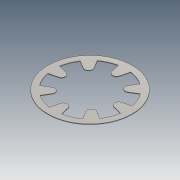
# Autodesk Inventor part: Arruela do parafuso da tampa
Saved by Autodesk Inventor 2016 (Build 200138000, 138)
## iProperties
Created: 2018-12-06
Part Number: Arruela do parafuso da tampa
Material: Generic
Document SubType Name: Modeling
Designer: Aluno
Density: 1 g/cm^3
Appearance: Galvanized
Author: Aluno
Autodesk Inventor part; units mm, degrees
ref_plane "YZ Plane" through (0, 0, 0) normal (1, 0, 0) x (0, 1, 0)
ref_plane "XZ Plane" through (0, 0, 0) normal (0, 1, 0) x (-1, 0, 0)
ref_plane "XY Plane" through (0, 0, 0) normal (0, 0, 1) x (1, 0, 0)
sketch "Sketch1" plane through (0, 0, 0) normal (0, 0, 1) x (1, 0, 0)
  circle A0 centre (0, 0) radius 7
  line L0 (0.1571, -3.914) -> (0.6571, -3.914)
  line L1 (0.6571, -3.914) -> (-0.3428, -3.914)
  line L2 (-0.3428, -3.914) -> (-0.8427, -5.9405)
  line L3 (0.6571, -3.914) -> (1.157, -5.8874)
  line L4 (2.5252, -3.01) -> (3.6047, -4.7964)
  line L5 (3.2322, -2.303) -> (4.9811, -3.3449)
  line L6 (2.8787, -2.6565) -> (3.2322, -2.303)
  line L7 (3.2322, -2.303) -> (2.5252, -3.01)
  line L8 (3.914, -0.3428) -> (5.9405, -0.8427)
  line L9 (3.914, 0.6571) -> (5.8874, 1.157)
  line L10 (3.914, 0.1571) -> (3.914, 0.6571)
  line L11 (3.914, 0.6571) -> (3.914, -0.3428)
  line L12 (3.01, 2.5252) -> (4.7964, 3.6047)
  line L13 (2.303, 3.2322) -> (3.3449, 4.9811)
  line L14 (2.6565, 2.8787) -> (2.303, 3.2322)
  line L15 (2.303, 3.2322) -> (3.01, 2.5252)
  line L16 (0.3428, 3.914) -> (0.8427, 5.9405)
  line L17 (-0.6571, 3.914) -> (-1.157, 5.8874)
  line L18 (-0.1571, 3.914) -> (-0.6571, 3.914)
  line L19 (-0.6571, 3.914) -> (0.3428, 3.914)
  line L20 (-2.5252, 3.01) -> (-3.6047, 4.7964)
  line L21 (-3.2322, 2.303) -> (-4.9811, 3.3449)
  line L22 (-2.8787, 2.6565) -> (-3.2322, 2.303)
  line L23 (-3.2322, 2.303) -> (-2.5252, 3.01)
  line L24 (-3.914, 0.3428) -> (-5.9405, 0.8427)
  line L25 (-3.914, -0.6571) -> (-5.8874, -1.157)
  line L26 (-3.914, -0.1571) -> (-3.914, -0.6571)
  line L27 (-3.914, -0.6571) -> (-3.914, 0.3428)
  line L28 (-3.01, -2.5252) -> (-4.7964, -3.6047)
  line L29 (-2.303, -3.2322) -> (-3.3449, -4.9811)
  line L30 (-2.6565, -2.8787) -> (-2.303, -3.2322)
  line L31 (-2.303, -3.2322) -> (-3.01, -2.5252)
  arc A1 (-4.9811, 3.3449) -> (-5.9405, 0.8427) centre (0, 0) ccw
  arc A2 (-1.157, 5.8874) -> (-3.6047, 4.7964) centre (0, 0) ccw
  arc A3 (3.3449, 4.9811) -> (0.8427, 5.9405) centre (0, 0) ccw
  arc A4 (5.8874, 1.157) -> (4.7964, 3.6047) centre (0, 0) ccw
  arc A5 (4.9811, -3.3449) -> (5.9405, -0.8427) centre (0, 0) ccw
  arc A6 (1.157, -5.8874) -> (3.6047, -4.7964) centre (0, 0) ccw
  arc A7 (-5.8874, -1.157) -> (-4.7964, -3.6047) centre (0, 0) ccw
  arc A8 (-3.3449, -4.9811) -> (-0.8427, -5.9405) centre (0, 0) ccw
  dimension "d7" = 360
  constraints: 64 end point, 16 point on circle, 9 centre point, 8 point on line, 1 coincident, 73 other
extrude "Extrusion1" add sketch "Sketch1" along normal blind 0.1
fillet "Fillet1" radius 0.65 16 edges at (-3.01, -2.5252, 0.05) (-2.303, -3.2322, 0.05) (-3.914, -0.6571, 0.05) (-3.914, 0.3428, 0.05) (0.6571, -3.914, 0.05) (-0.3428, -3.914, 0.05) (-0.6571, 3.914, 0.05) (0.3428, 3.914, 0.05) (2.5252, -3.01, 0.05) (3.2322, -2.303, 0.05) (3.914, 0.6571, 0.05) (3.914, -0.3428, 0.05) (2.303, 3.2322, 0.05) (3.01, 2.5252, 0.05) (-3.2322, 2.303, 0.05) (-2.5252, 3.01, 0.05)
body "Solid1"
